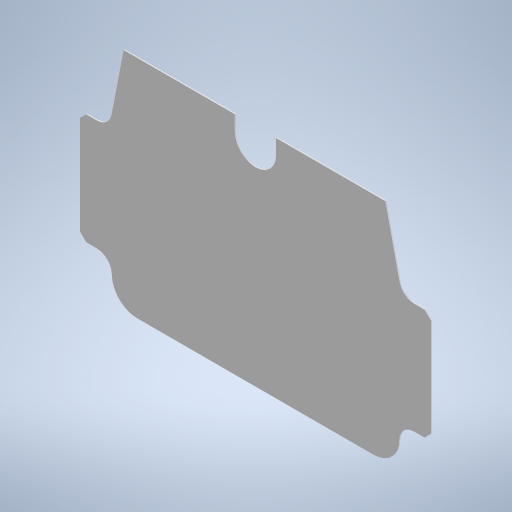
# Autodesk Inventor part: Součást5
Saved by Autodesk Inventor 2024 (Build 280153000, 153)
## iProperties
Created: 2023-11-14
Part Number: Součást5
Material: Všeobecné
Document SubType Name: Modeling
Designer: Simak
Density: 1 g/cm^3
Appearance: Výchozí
Author: Simak
Autodesk Inventor part; units mm, degrees
ref_plane "YZ Plane" through (0, 0, 0) normal (1, 0, 0) x (0, 1, 0)
ref_plane "XZ Plane" through (0, 0, 0) normal (0, 1, 0) x (-1, 0, 0)
ref_plane "XY Plane" through (0, 0, 0) normal (0, 0, 1) x (1, 0, 0)
sketch "Náčrt1" plane through (0, 0, 0) normal (0, 0, 1) x (1, 0, 0)
  line L0 (49.75, 43.4103) -> (-49.75, 43.4103) projected
  line L1 (-49.75, 43.4103) -> (-49.75, -24.25) projected
  line L2 (-49.75, -24.25) -> (-27, -24.25) projected
  line L3 (-27, -24.25) -> (-27, -44.75) projected
  line L4 (-27, -44.75) -> (-5, -44.75) projected
  line L5 (-5, -44.75) -> (-5, -40.875) projected
  arc A0 (5, -40.875) -> (-5, -40.875) centre (0, -40.875) ccw projected
  line L6 (5, -40.875) -> (5, -44.75) projected
  line L7 (5, -44.75) -> (27, -44.75) projected
  line L8 (27, -44.75) -> (27, -24.25) projected
  line L9 (27, -24.25) -> (49.75, -24.25) projected
  line L10 (49.75, -24.25) -> (49.75, 43.4103) projected
  circle A1 centre (22, -29.1875) radius 1.75 projected
  circle A2 centre (-22, -29.1875) radius 1.75 projected
  circle A3 centre (-42.25, -13.5) radius 1.75 projected
  circle A4 centre (-42.25, 24) radius 1.75 projected
  circle A5 centre (42.25, 24) radius 1.75 projected
  circle A6 centre (42.25, -13.5) radius 1.75 projected
  circle A7 centre (41.136, 35.833) radius 5 projected
  circle A8 centre (-41.463, 35.833) radius 5 projected
  circle A9 centre (0, 35.833) radius 5 projected
  line L11 (49.75, 43.4103) -> (-49.75, 43.4103) projected
  line L12 (-49.75, 43.4103) -> (-49.75, -24.25) projected
  line L13 (-49.75, -24.25) -> (-27, -24.25) projected
  line L14 (-27, -24.25) -> (-27, -44.75) projected
  line L15 (-27, -44.75) -> (-5, -44.75) projected
  line L16 (-5, -44.75) -> (-5, -40.875) projected
  arc A10 (5, -40.875) -> (-5, -40.875) centre (0, -40.875) ccw projected
  line L17 (5, -40.875) -> (5, -44.75) projected
  line L18 (5, -44.75) -> (27, -44.75) projected
  line L19 (27, -44.75) -> (27, -24.25) projected
  line L20 (27, -24.25) -> (49.75, -24.25) projected
  line L21 (49.75, -24.25) -> (49.75, 43.4103) projected
  circle A11 centre (22, -29.1875) radius 1.75 projected
  circle A12 centre (-22, -29.1875) radius 1.75 projected
  circle A13 centre (-42.25, -13.5) radius 1.75 projected
  circle A14 centre (-42.25, 24) radius 1.75 projected
  circle A15 centre (42.25, 24) radius 1.75 projected
  circle A16 centre (42.25, -13.5) radius 1.75 projected
  circle A17 centre (41.136, 35.833) radius 5 projected
  circle A18 centre (-41.463, 35.833) radius 5 projected
  circle A19 centre (0, 35.833) radius 5 projected
  line L22 (49.75, 43.4103) -> (-49.75, 43.4103) projected
  line L23 (-49.75, 43.4103) -> (-49.75, -24.25) projected
  line L24 (-49.75, -24.25) -> (-27, -24.25) projected
  line L25 (-27, -24.25) -> (-27, -44.75) projected
  line L26 (-27, -44.75) -> (-5, -44.75) projected
  line L27 (-5, -44.75) -> (-5, -40.875) projected
  arc A20 (5, -40.875) -> (-5, -40.875) centre (0, -40.875) ccw projected
  line L28 (5, -40.875) -> (5, -44.75) projected
  line L29 (5, -44.75) -> (27, -44.75) projected
  line L30 (27, -44.75) -> (27, -24.25) projected
  line L31 (27, -24.25) -> (49.75, -24.25) projected
  line L32 (49.75, -24.25) -> (49.75, 43.4103) projected
  circle A21 centre (22, -29.1875) radius 1.75 projected
  circle A22 centre (-22, -29.1875) radius 1.75 projected
  circle A23 centre (-42.25, -13.5) radius 1.75 projected
  circle A24 centre (-42.25, 24) radius 1.75 projected
  circle A25 centre (42.25, 24) radius 1.75 projected
  circle A26 centre (42.25, -13.5) radius 1.75 projected
  circle A27 centre (41.136, 35.833) radius 5 projected
  circle A28 centre (-41.463, 35.833) radius 5 projected
  circle A29 centre (0, 35.833) radius 5 projected
  arc A30 (23.3253, -53.0519) -> (20.6747, -53.0519) centre (22, -49.8125) ccw projected
  line L33 (0.0392, -53.0519) -> (20.6747, -53.0519) projected
  line L34 (2.825, -51.4435) -> (0.0392, -53.0519) projected
  line L35 (2.825, -48.1815) -> (2.825, -51.4435) projected
  line L36 (0, -46.5505) -> (2.825, -48.1815) projected
  line L37 (-2.825, -48.1815) -> (0, -46.5505) projected
  line L38 (-2.825, -51.4435) -> (-2.825, -48.1815) projected
  line L39 (-0.0392, -53.0519) -> (-2.825, -51.4435) projected
  line L40 (-20.6747, -53.0519) -> (-0.0392, -53.0519) projected
  arc A31 (-20.6747, -53.0519) -> (-23.3253, -53.0519) centre (-22, -49.8125) ccw projected
  line L41 (-27, -53.0519) -> (-23.3253, -53.0519) projected
  line L42 (-27, -24.25) -> (-27, -53.0519) projected
  line L43 (-49.75, -24.25) -> (-27, -24.25) projected
  line L44 (-49.75, 43.4103) -> (-49.75, -24.25) projected
  line L45 (49.75, 43.4103) -> (-49.75, 43.4103) projected
  line L46 (49.75, -24.25) -> (49.75, 43.4103) projected
  line L47 (27, -24.25) -> (49.75, -24.25) projected
  line L48 (27, -53.0519) -> (27, -24.25) projected
  line L49 (23.3253, -53.0519) -> (27, -53.0519) projected
  circle A32 centre (22, -29.1875) radius 1.85 projected
  circle A33 centre (-22, -29.1875) radius 1.85 projected
  circle A34 centre (42.25, -13.5) radius 1.85 projected
  circle A35 centre (42.25, 24) radius 1.85 projected
  circle A36 centre (-42.25, -13.5) radius 1.85 projected
  circle A37 centre (-42.25, 24) radius 1.85 projected
  arc A38 (42.25, -10) -> (38.75, -13.5) centre (42.25, -13.5) ccw projected
  line L50 (45.25, -10) -> (42.25, -10) projected
  line L51 (47.25, -8) -> (45.25, -10) projected
  line L52 (47.25, 18.5) -> (47.25, -8) projected
  line L53 (45.25, 20.5) -> (47.25, 18.5) projected
  line L54 (42.25, 20.5) -> (45.25, 20.5) projected
  arc A39 (42.25, 27.5) -> (42.25, 20.5) centre (42.25, 24) ccw projected
  line L55 (45.25, 27.5) -> (42.25, 27.5) projected
  line L56 (47.25, 29.5) -> (45.25, 27.5) projected
  line L57 (47.25, 40.3044) -> (47.25, 29.5) projected
  line L58 (-47.25, 40.3044) -> (47.25, 40.3044) projected
  line L59 (-47.25, 29.5) -> (-47.25, 40.3044) projected
  line L60 (-45.25, 27.5) -> (-47.25, 29.5) projected
  line L61 (-42.25, 27.5) -> (-45.25, 27.5) projected
  arc A40 (-42.25, 20.5) -> (-42.25, 27.5) centre (-42.25, 24) ccw projected
  line L62 (-45.25, 20.5) -> (-42.25, 20.5) projected
  line L63 (-47.25, 18.5) -> (-45.25, 20.5) projected
  line L64 (-47.25, -8) -> (-47.25, 18.5) projected
  line L65 (-45.25, -10) -> (-47.25, -8) projected
  line L66 (-42.25, -10) -> (-45.25, -10) projected
  arc A41 (-38.75, -13.5) -> (-42.25, -10) centre (-42.25, -13.5) ccw projected
  arc A42 (-38.75, -13.5) -> (-31.5, -20.75) centre (-31.5, -13.5) ccw projected
  line L67 (-31.5, -20.75) -> (31.5, -20.75) projected
  arc A43 (31.5, -20.75) -> (38.75, -13.5) centre (31.5, -13.5) ccw projected
  line L68 (5, -46.375) -> (5, -40.875) projected
  arc A44 (5, -40.875) -> (-5, -40.875) centre (0, -40.875) ccw projected
  line L69 (-5, -46.375) -> (-5, -40.875) projected
  line L70 (-5, -46.375) -> (5, -46.375) projected
  line L71 (-38.8151, 23.3279) -> (-35.4932, 40.3044)
  line L72 (38.8347, 23.2348) -> (35.0102, 40.3044)
  line L73 (-5, 35.833) -> (-5, 40.3044)
  line L74 (5, 35.833) -> (5, 40.3044)
  line L75 (-42.25, 28) -> (-45.0429, 28)
  line L76 (-45.0429, 28) -> (-46.75, 29.7071)
  line L77 (-46.75, 29.7071) -> (-46.75, 39.8044)
  line L78 (-46.75, 39.8044) -> (46.75, 39.8044)
  line L79 (46.75, 39.8044) -> (46.75, 29.7071)
  line L80 (46.75, 29.7071) -> (45.0429, 28)
  line L81 (45.0429, 28) -> (42.25, 28)
  arc A45 (42.25, 28) -> (42.25, 20) centre (42.25, 24) ccw
  line L82 (42.25, 20) -> (45.0429, 20)
  line L83 (45.0429, 20) -> (46.75, 18.2929)
  line L84 (46.75, 18.2929) -> (46.75, -7.7929)
  line L85 (46.75, -7.7929) -> (45.0429, -9.5)
  line L86 (45.0429, -9.5) -> (42.25, -9.5)
  arc A46 (42.25, -9.5) -> (38.25, -13.5) centre (42.25, -13.5) ccw
  arc A47 (31.5, -20.25) -> (38.25, -13.5) centre (31.5, -13.5) ccw
  line L87 (31.5, -20.25) -> (-31.5, -20.25)
  arc A48 (-38.25, -13.5) -> (-31.5, -20.25) centre (-31.5, -13.5) ccw
  arc A49 (-38.25, -13.5) -> (-42.25, -9.5) centre (-42.25, -13.5) ccw
  line L88 (-42.25, -9.5) -> (-45.0429, -9.5)
  line L89 (-45.0429, -9.5) -> (-46.75, -7.7929)
  line L90 (-46.75, -7.7929) -> (-46.75, 18.2929)
  line L91 (-46.75, 18.2929) -> (-45.0429, 20)
  line L92 (-45.0429, 20) -> (-42.25, 20)
  arc A50 (-42.25, 20) -> (-42.25, 28) centre (-42.25, 24) ccw
  line L93 (-38.3244, 23.2319) -> (-35.0025, 40.2084)
  line L94 (38.3468, 23.1255) -> (34.5223, 40.1951)
  circle A51 centre (0, 35.833) radius 5.5
  line L95 (5.5, 35.833) -> (5.5, 40.3044)
  line L96 (-5.5, 35.833) -> (-5.5, 40.3044)
  point P0 (0, 0)
  point P1 (34.6098, 39.8044)
  point P2 (5.5, 39.8044)
  point P3 (5.5, 35.833)
  point P4 (-5.5, 39.8044)
  point P5 (-35.0816, 39.8044)
  dimension "d1" = 0.5
  dimension "d2" = 0.5
  dimension "d3" = 0.5
  dimension "d4" = 0.5
  dimension "d5" = 0.5
  dimension "d6" = 0.5
  constraints: 52 end point, 16 point on circle, 10 tangent, 7 centre point, 4 parallel, 4 point on line, 1 perpendicular, 1 vertical, 23 other
  measures "d1" radial gap between concentric circles of A40 A50
  measures "d2" distance between parallel lines of L71 L93
  measures "d3" distance between parallel lines of L72 L94
  measures "d4" radial gap between concentric circles of A9 A51
  measures "d5" distance between parallel lines of L74 L95
  measures "d6" distance between parallel lines of L73 L96
extrude "Vysunutí1" add sketch "Náčrt1" along normal blind 0.3 contours A45 L82 L83 L84 L85 L86 A46 A47 L87 A48 A49 L88 L89 L90 L91 L92 A50 L93 L78 L96 A51 L95 L94
